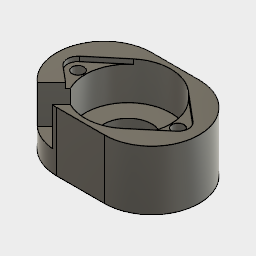
motor drill jig (Autodesk Fusion 360 design; units mm, degrees)
Autodesk Fusion 360 part; units mm, degrees
box "BoxPrimitive1" add length 40 width 60 height 25 placed x (0, 0, -1) y (-1, 0, 0) z (0, 1, 0) at (30, 0, 20)
cylinder "CylinderPrimitive1" cut diameter 36 height -16 placed x (1, 0, 0) y (0, 0, -1) z (0, 1, 0) at (0, 25, 0)
hole "Hole1" at (0, 9, 0) direction (0, -1, 0) diameter 20 depth 17 tip angle 118
sketch "Sketch4" plane through (0, 25, 0) normal (0, 1, 0) x (-1, 0, 0)
  circle A0 centre (0, 0) radius 18
  line L0 (-30, -20) -> (30, -20)
  line L1 (30, -20) -> (30, 20)
  line L2 (30, 20) -> (-30, 20)
  line L3 (-30, 20) -> (-30, -20)
  arc A1 (23.8929, -3.4469) -> (23.8929, 3.4469) centre (21, 0) ccw
  arc A2 (-23.8929, 3.4469) -> (-23.8929, -3.4469) centre (-21, 0) ccw
  arc A3 (-11.5714, -13.7877) -> (11.5714, -13.7877) centre (0, 0) ccw
  arc A4 (11.5714, 13.7877) -> (-11.5714, 13.7877) centre (0, 0) ccw
  line L4 (23.8929, -3.4469) -> (11.5714, -13.7877)
  line L5 (-11.5714, -13.7877) -> (-23.8929, -3.4469)
  line L6 (-23.8929, 3.4469) -> (-11.5714, 13.7877)
  line L7 (11.5714, 13.7877) -> (23.8929, 3.4469)
  dimension "d11" = 4.5
  dimension "d12" = 4.5
  dimension "d13" = 21
  dimension "d14" = 21
  measures "d11" radius of A2
  measures "d12" radius of A1
  measures "d13" distance of A0.centre A1.centre
  measures "d14" distance of A0.centre A2.centre
extrude "Extrude1" cut sketch "Sketch4" against normal blind 2 contours A0 A1 L4 L7 | A0 A2 L5 L6
hole "Hole2" at (-21, 23, 0) direction (0, -1, 0) diameter 5 end through all
hole "Hole3" at (21, 23, 0) direction (0, -1, 0) diameter 5 end through all
fillet "Fillet1" radius 20 1 edges at (-30, 12.5, 20)
fillet "Fillet1" radius 20 3 edges at (30, 12.5, 20) (30, 12.5, -20) (-30, 12.5, -20)
sketch "Sketch5" plane through (0, 25, 0) normal (0, 1, 0) x (-1, 0, 0)
  arc A0 (10, -20) -> (10, 20) centre (10, 0) ccw
  line L0 (10, 20) -> (-10, 20)
  arc A1 (-10, 20) -> (-10, -20) centre (-10, 0) ccw
  line L1 (-10, -20) -> (10, -20)
  line L2 (23.8929, -3.4469) -> (11.5714, -13.7877)
  arc A2 (-11.5714, -13.7877) -> (11.5714, -13.7877) centre (0, 0) ccw
  line L3 (-11.5714, -13.7877) -> (-23.8929, -3.4469)
  arc A3 (-23.8929, 3.4469) -> (-23.8929, -3.4469) centre (-21, 0) ccw
  line L4 (-23.8929, 3.4469) -> (-11.5714, 13.7877)
  arc A4 (11.5714, 13.7877) -> (-11.5714, 13.7877) centre (0, 0) ccw
  line L5 (11.5714, 13.7877) -> (23.8929, 3.4469)
  arc A5 (23.8929, -3.4469) -> (23.8929, 3.4469) centre (21, 0) ccw
  line L6 (8, 0) -> (0, 8)
  line L7 (0, 8) -> (20.2173, 28.2173)
  line L8 (20.2173, 28.2173) -> (28.2173, 20.2173)
  line L9 (28.2173, 20.2173) -> (8, 0)
  dimension "d25" = 8
  dimension "d26" = 8
  measures "d25" distance of A2.centre L6.end
  measures "d26" distance of A2.centre L6.start
extrude "Extrude2" cut sketch "Sketch5" against normal blind 16 contours A0 A4 L5 L7 L9 | A0 L7 L8 L9 | A4 L5 L6 L7 L9
equation "d13 = ( 42 / 2 ) * 1 mm"
equation "d14 = ( 42 / 2 ) * 1 mm"
